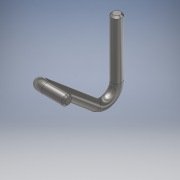
# Autodesk Inventor part: Barre
Saved by Autodesk Inventor 2017 (Build 210142000, 142)
## iProperties
Company: FABLAB Frenchmakers
Part Number: Barre
Material: Acier inoxydable
Document SubType Name: Modeling
Designer: FABLAB Frenchmakers
Density: 8 g/cm^3
Appearance: Semi-poli
Mass: 26.7098 g
Surface Area: 22.6885 cm^2
Volume: 3.33873 cm^3
Project: 1400-PopCorn Machine
Stock Number: 1400-01-07
Author: Adrien MARY
Autodesk Inventor part; units mm, degrees
ref_plane "YZ Plane" through (0, 0, 0) normal (1, 0, 0) x (0, 1, 0)
ref_plane "XZ Plane" through (0, 0, 0) normal (0, 1, 0) x (-1, 0, 0)
ref_plane "XY Plane" through (0, 0, 0) normal (0, 0, 1) x (1, 0, 0)
sketch "Esquisse4" plane through (0, 0, 0) normal (0, 0, 1) x (1, 0, 0)
  circle A0 centre (0, 0) radius 3
  dimension "d15" = 6
  constraints: 1 centre point, 1 coincident
  measures "d15" diameter of A0
sketch3d "Esquisse 3D1"
  line L0 (0, 0, 0) -> (0, 0, -34.8439)
  arc A0 (0, 0, -34.8439) -> (0, -13.1423, -40.9723) centre (0, -8, -34.8439) ccw
  line L1 (0, -13.1423, -40.9723) -> (0, -43.8716, -15.1873)
  arc A1 (0, -43.8716, -15.1873) -> (8, -50, -10.045) centre (8, -43.8716, -15.1873) ccw
  line L2 (8, -50, -10.045) -> (21, -50, -10.045)
  dimension "d11" = 52
  dimension "d12" = 21
  dimension "d13" = 8
  dimension "d14" = 8
  constraints: 2 horizontal
sweep "Balayage2" add profiles "Esquisse4" path "Esquisse 3D1"
chamfer "Chanfrein1" distance 1 angle 45 6 edges at (-3, 0, 0) (-3, 0, -34.8439) (-3, -13.1423, -40.9723) (-3, -43.8716, -15.1873) (8, -52.2981, -8.1167) (21, -52.2981, -8.1167)
equation "\"nombredor\" = 1.61803"
equation "\"pi\" = 3.141593"
